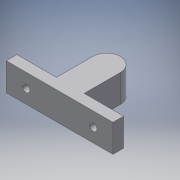
# Autodesk Inventor part: Z-Gevind-Holder
Saved by Autodesk Inventor 2016 SP1 (Build 200210100, 210)
## iProperties
Created: 2015-06-08
Part Number: Z-Gevind-Holder
Material: PC/ABS Plastic
Document SubType Name: Modeling
Designer: Mathias L. Kjeldgaard
Mass: 7.95438 g
Surface Area: 79.3155 cm^2
Volume: 22.2642 cm^3
Density: 0.357273 g/cm^3
Appearance: Smooth - White
Author: Mathias L. Kjeldgaard
Autodesk Inventor part; units mm, degrees
ref_plane "YZ Plane" through (0, 0, 0) normal (1, 0, 0) x (0, 1, 0)
ref_plane "XZ Plane" through (0, 0, 0) normal (0, 1, 0) x (-1, 0, 0)
sketch "Sketch1" plane through (0, 0, 0) normal (0, 0, 1) x (1, 0, 0)
  circle A0 centre (0, 11) radius 4 construction
  circle A1 centre (0, 11) radius 4.5
  line L0 (200.3677, 25.2343) -> (-185.7345, -79.2887) construction
  line L1 (200.3677, 25.2343) -> (210.1768, -11) construction
  line L2 (-204.2212, -11) -> (210.1768, -11) construction
  line L3 (-185.7345, -79.2887) -> (-204.2212, -11) construction
  arc A2 (6.5, 11) -> (-6.5, 11) centre (0, 11) ccw
  line L4 (6.5, 11) -> (6.5, -6)
  line L5 (-6.5, 11) -> (-6.5, -6)
  line L6 (25, -6) -> (25, -11)
  line L7 (-25, -6) -> (-25, -11)
  line L8 (-25, -11) -> (25, -11)
  line L9 (-25, -6) -> (-6.5, -6)
  line L10 (6.5, -6) -> (25, -6)
  point P0 (0, 0)
  dimension "d0" = 0.5
  dimension "d1" = 2
  dimension "d3" = 18.5
  dimension "d4" = 13
  dimension "d5" = 18.5
  dimension "d6" = 5
  dimension "d7" = 5
  dimension "d20" = 22
  dimension "d21" = 11
  dimension "d22" = 25
  dimension "d23" = 50
  constraints: 22 end point, 6 perpendicular, 3 centre point, 2 coincident, 2 point on circle, 2 point on line, 2 tangent, 1 collinear, 1 horizontal
  measures "d0" radial gap between concentric circles of A1 A0
  measures "d1" radial gap between concentric circles of A2 A1
  measures "d3" distance between parallel lines of L4 L6
  measures "d4" distance between parallel lines of L5 L4
  measures "d5" distance between parallel lines of L5 L7
  measures "d6" distance between parallel lines of L8 L10
  measures "d7" distance between parallel lines of L8 L9
  measures "d20" distance from line of A0.centre L8
  measures "d21" distance from line of point (0, 0) L8
  measures "d22" distance from line of point (0, 0) L6
  measures "d23" distance between parallel lines of L7 L6
ref_plane "Work Plane1" through (-2, -2, 20) normal (0, 0, 1) x (1, 0, 0)
extrude "Tykkelse" add sketch "Sketch1" along normal blind 13
sketch "Sketch2" plane through (-25, -11, 0) normal (0, -1, 0) x (1, 0, 0)
  line L0 (0, 13) -> (50, 13) projected
  line L1 (0, 0) -> (0, 13) projected
  line L2 (18.5, 0) -> (0, 0) projected
  line L3 (0, 0) -> (0, 13) projected
  line L4 (18.5, 13) -> (0, 13) projected
  line L5 (18.5, 0) -> (18.5, 13) projected
  line L6 (50, 0) -> (31.5, 0) projected
  line L7 (31.5, 0) -> (31.5, 13) projected
  line L8 (50, 13) -> (31.5, 13) projected
  line L9 (50, 0) -> (50, 13) projected
  circle A0 centre (9.25, 6.5) radius 1.75
  circle A1 centre (40.75, 6.5) radius 1.75
  point P0 (25, 0)
  dimension "d10" = 3.5
  dimension "d11" = 3.5
  dimension "d12" = 9.25
  dimension "d13" = 9.25
  dimension "d14" = 6.5
  dimension "d15" = 6.5
  dimension "d16" = 9.25
  dimension "d17" = 6.5
  constraints: 2 centre point
  measures "d10" diameter of A0
  measures "d11" diameter of A1
  measures "d12" distance from line of L5 A0.centre
  measures "d13" distance from line of L1 A0.centre
  measures "d14" distance from line of L0 A0.centre
  measures "d15" distance from line of L2 A0.centre
  measures "d16" distance from line of L9 A1.centre
  measures "d17" distance from line of L0 A1.centre
extrude "Monteringshuller" cut sketch "Sketch2" against normal up to surface (5 mm away) contours A0 | A1
sketch "Sketch3" plane through (0, 0, 13) normal (0, 0, 1) x (1, 0, 0)
  circle A0 centre (0, 11) radius 4.5 construction
  arc A1 (6.5, 11) -> (-6.5, 11) centre (0, 11) ccw construction
  line L0 (-6.5, 11) -> (-6.5, -6) construction
  line L1 (-6.5, -6) -> (-25, -6) construction
  line L2 (-25, -6) -> (-25, -11) construction
  line L3 (-25, -11) -> (25, -11) construction
  line L4 (25, -11) -> (25, -6) construction
  line L5 (25, -6) -> (6.5, -6) construction
  line L6 (6.5, -6) -> (6.5, 11) construction
  circle A2 centre (0, 11) radius 4.5
  point P0 (0, 0)
  constraints: 1 centre point, 1 coincident
extrude "Fyld hul" add sketch "Sketch3" against normal blind 2
equation "\"d5\" = d3"
equation "\"d7\" = d6"
equation "\"d21\" = 0.5 * d20"
equation "\"d22\" = 0.5 * d23"
equation "\"d11\" = d10"
equation "\"d12\" = d13"
equation "\"d14\" = d15"
equation "\"d16\" = d12"
equation "\"d17\" = d14"
body "Solid1"
